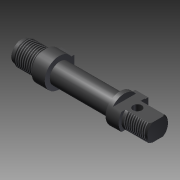
# Autodesk Inventor part: 16N2A12A010-(N0-cilindro)
Saved by Autodesk Inventor 2011 SP1 (Build 150282100, 282)
## iProperties
Created: 2018-01-08
Part Number: 16N2A12A010-(N0-cilindro)
Catalog Web Link: www.cadenas.de
Description: Minicylinders Serie 16 - 24 - 25 Single and double acting  Cetop RP52-P DIN/ISO 6432-Cylinder-
Vendor: CAMOZZI
Document SubType Name: Modeling
Designer: psAdmin
Manufacturer: CAMOZZI
Mass: 14.7107 g
Surface Area: 75.8728 cm^2
Volume: 14.7107 cm^3
Density: 1 g/cm^3
Category: PARTsolutions
Company: CAMOZZI
Title: 16N2A12A010
Author: Cadenas PARTsolutions
PSOL_IDENT_0: {$CADENAS_DATA\23d-libs\camozzi\movimento\cilindri_a_norma_e_cilindri_standard\minicilindri_serie_16
PSOL_IDENT_1: _24_25\minicilindr_serie_16_24_25_cilindro.prj},289 {VTYP=3D},{NB=16N2A12A010-(N0-cilindro)},{LINA=1
PSOL_IDENT_2: 6N2A12A010},{NN=Minicylinders Serie 16 - 24 - 25 Single and double acting  Cetop RP52-P DIN/ISO 6432
PSOL_IDENT_3: -Cylinder},{DATE=27.07.2017 08:45:31},{GEOMDATE=02.04.2015 14:04:54},{VERSION=},{LINEID=40},{LINESUB
PSOL_IDENT_4: ID=-1},{WBVAR=FUNZ,HUBT,HUB,TYP,LSTELO}  {NB=16N2A12A010-(N0-cilindro)},{LINA=16N2A12A010},{KT=DUMMY
PSOL_IDENT_5: },{IDNR=},{SERIE=16},{PHY=12},{EW=12},{KW=8},{BE=M16x1.5},{BENDM=16.000},{BEKDM=14.160},{KK=M6x1},{K
PSOL_IDENT_6: KNDM=6.000},{KKDM=4.773},{CD=6},{VERSION=N = standard},{FUNZ=2},{HUBT=N},{HUB=10},{MAT=A = stelo INO
PSOL_IDENT_7: X rullato - camicia inox},{TYP=A},{V=V = guarnizione stelo viton},{LSTELO=0},{LSTELOX=[0-1000]},{D1=
PSOL_IDENT_8: 14.0},{EE=M5},{EENDM=5.000},{EEKDM=4.019},{D2=6},{L1=105.0},{L11=105.0},{L12=126.0},{L13=0.000},{XC=
PSOL_IDENT_9: 75},{XC1=75},{XC2=0.000},{L2=50.0},{AM=16},{L3=15},{L4=4.5},{L5=17},{L5X1=17},{L5X2=0.000},{L=9},{WF=
PSOL_IDENT_10: 22},{WF1=22},{WF2=0.000},{L6=9},{L7=38},{L7X1=38},{L7X2=0.000},{KV=24},{SW=5},{D=20.5},{D3=20},{HUBA=
PSOL_IDENT_11: -},{FIN=1,'1=semplice effetto',2,'2=doppio effetto',3,'3=doppio effetto stelo passante',7,'7=s.e. st
PSOL_IDENT_12: elo passante'},{HUBIN=10,25,40,50,80,100,125,160,200,250,300},{HUBIN1=10,25,40,50},{HUBIN2=[10:50]},
PSOL_IDENT_13: {HUBIN3=10,25,40,50,80,100,125,160,200,250,300},{HUBIN4=[10:300]},{TYPIN1= 'A', 'A=ghiera V + dado s
PSOL_IDENT_14: telo U'},{TYPIN2= 'A', 'A=ghiera V + dado stelo U'},{TYPIN= 'A', 'A=ghiera V + dado stelo U'},{L51=2
PSOL_IDENT_15: .000},{PRA=1},{HUBX=010},{PHYX=12},{XS=0.000},{YS=0.000},{TB=0.000},{TS=0.000},{DS=0.000}
NN: Minicylinders Serie 16 - 24 - 25 Single and double acting  Cetop RP52-P DIN/ISO 6432-Cylinder
NB: 16N2A12A010-(N0-cilindro)
NBSYN: $SERIE.N$FUNZ.A$PHYX.$TYP.$HUBX.-($HUBT.$LSTELO.-cilindro)
LINA: 16N2A12A010
SERIE: 16
PHY: 12
EW: 12
KW: 8
BE: M16x1.5
KK: M6x1
CD: 6
VERSION: N = standard
FUNZ: 2=doppio effetto
HUBT: standard
HUB: 10
MAT: A = stelo INOX rullato - camicia inox
TYP: A=ghiera V + dado stelo U
V: V = guarnizione stelo viton
LSTELO: 0
D1: 14.0
EE: M5
D2: 6
L1: 105.0
L13: 0.000
XC1: 75
XC2: 0.000
L2: 50.0
AM: 16
L3: 15
L4: 4.5
L5X1: 17
L5X2: 0.000
L: 9
WF1: 22
WF2: 0.000
L6: 9
L7X1: 38
L7X2: 0.000
KV: 24
SW: 5
D: 20.5
D3: 20
HUBA: -
TYPIN1: 'A', 'A=ghiera V + dado stelo U'
TYPIN2: 'A', 'A=ghiera V + dado stelo U'
L51: 2.000
XS: 0.000
YS: 0.000
TB: 0.000
TS: 0.000
DS: 0.000
SUPPLIER: CAMOZZI
ARTICLENO: 16N2A12A010-(N0-cilindro)
BOMINFO: 16N2A12A010
CREATOR: CADENAS GmbH
Autodesk Inventor part; units mm, degrees
sketch "Skizze_1" plane through (0, 0, 0) normal (0, 0, 1) x (1, 0, 0)
  line L0 (77, 0) -> (-17, 0)
  line L1 (-17, 0) -> (-17, 7.08)
  line L2 (-17, 7.08) -> (-15, 7.08)
  line L3 (-15, 7.08) -> (-14.08, 8)
  line L4 (-14.08, 8) -> (0, 8)
  line L5 (0, 8) -> (0, 10)
  line L6 (0, 10) -> (9, 10)
  line L7 (9, 10) -> (9, 6.5)
  line L8 (9, 6.5) -> (9.5, 7)
  line L9 (9.5, 7) -> (50.5, 7)
  line L10 (50.5, 7) -> (51, 6.5)
  line L11 (51, 6.5) -> (51, 10)
  line L12 (51, 10) -> (60, 10)
  line L13 (60, 10) -> (60, 8)
  line L14 (60, 8) -> (76.08, 8)
  line L15 (76.08, 8) -> (77, 7.08)
  line L16 (77, 7.08) -> (77, 0)
  line L17 (77, 0) -> (-17, 0)
  constraints: 36 end point
revolve "Revolution1" add sketch "Skizze_1" angle 360 about axis through (77, 0, 0) along (1, 0, 0)
thread "Thread1" size "M16x1.5" class "6g" standard "ISO Metric profile" length 12.08
thread "Thread2" size "M16x1.5" class "6g" standard "ISO Metric profile" length 14.4865
sketch "Skizze_3" plane through (0, 0, 0) normal (1, 0, 0) x (0, 1, 0)
  line L0 (10.5, 5.5) -> (0, 5.5)
  line L1 (0, 5.5) -> (0, -5.5)
  line L2 (0, -5.5) -> (10.5, -5.5)
  line L3 (10.5, -5.5) -> (10.5, 5.5)
  constraints: 8 end point
extrude "Extrusion1" add sketch "Skizze_3" along normal blind 9
sketch "Skizze_4" plane through (60, 0, 0) normal (1, 0, 0) x (0, 0, -1)
  line L0 (-5.5, 10.5) -> (-5.5, 0)
  line L1 (-5.5, 0) -> (5.5, 0)
  line L2 (5.5, 0) -> (5.5, 10.5)
  line L3 (5.5, 10.5) -> (-5.5, 10.5)
  constraints: 8 end point
extrude "Extrusion2" add sketch "Skizze_4" against normal blind 9
sketch "Skizze_16_ALT_Drilling_1" plane through (0, 0, 0) normal (0, 0, 1) x (1, 0, 0)
  line L0 (51, 0) -> (-17, 0)
  line L1 (-17, 0) -> (-17, 3)
  line L2 (-17, 3) -> (38, 3)
  line L3 (38, 3) -> (38, 5.6)
  line L4 (38, 5.6) -> (51, 5.6)
  line L5 (51, 5.6) -> (51, 0)
  line L6 (51, 0) -> (-17, 0)
  constraints: 14 end point
revolve "Revolution2" cut sketch "Skizze_16_ALT_Drilling_1" angle 360 about axis through (51, 0, 0) along (1, 0, 0)
sketch "Skizze_7" plane through (0, 0, 0) normal (0, 1, 0) x (-1, 0, 0)
  line L0 (-54, -12) -> (-54, -6)
  line L1 (-54, -6) -> (-77, -6)
  line L2 (-77, -6) -> (-77, 6)
  line L3 (-77, 6) -> (-54, 6)
  line L4 (-54, 6) -> (-54, 12)
  line L5 (-54, 12) -> (-86, 12)
  line L6 (-86, 12) -> (-86, -12)
  line L7 (-86, -12) -> (-54, -12)
  constraints: 16 end point
extrude "Extrusion3" cut sketch "Skizze_7" along normal mid plane 24
sketch "Skizze_8" plane through (0, 0, 0) normal (0, 0, 1) x (1, 0, 0)
  circle A0 centre (63, 0) radius 3
  constraints: 1 centre point
extrude "Extrusion4" cut sketch "Skizze_8" along normal mid plane 24
sketch "Skizze_9_ALT_Drilling_2" plane through (0, 0, 0) normal (0, 0, 1) x (1, 0, 0)
  line L0 (4.5, 10.5) -> (4.5, 5.3398)
  line L1 (4.5, 5.3398) -> (2.4905, 6.5)
  line L2 (2.4905, 6.5) -> (2.4905, 10.0095)
  line L3 (2.4905, 10.0095) -> (2, 10.5)
  line L4 (2, 10.5) -> (4.5, 10.5)
  line L5 (4.5, 10.5) -> (4.5, 5.3398)
  constraints: 12 end point
revolve "Revolution3" cut sketch "Skizze_9_ALT_Drilling_2" angle 360 about axis through (4.5, 10.5, 0) along (0, 1, 0)
sketch "Skizze_10_ALT_Drilling_3" plane through (0, 0, 0) normal (0, 0, 1) x (1, 0, 0)
  line L0 (55.5, 10.5) -> (55.5, 5.3398)
  line L1 (55.5, 5.3398) -> (53.4905, 6.5)
  line L2 (53.4905, 6.5) -> (53.4905, 10.0095)
  line L3 (53.4905, 10.0095) -> (53, 10.5)
  line L4 (53, 10.5) -> (55.5, 10.5)
  line L5 (55.5, 10.5) -> (55.5, 5.3398)
  constraints: 12 end point
revolve "Revolution4" cut sketch "Skizze_10_ALT_Drilling_3" angle 360 about axis through (55.5, 10.5, 0) along (0, 1, 0)
ref_plane "C1_XY" through (0, 0, 0) normal (1, 0, 0) x (0, 0, -1)
ref_plane "C1_YZ" through (0, 0, 0) normal (0, 0, -1) x (0, 1, 0)
ref_plane "C1_ZX" through (0, 0, 0) normal (0, 1, 0) x (1, 0, 0)
ref_plane "CD1_XY" through (0, 0, 0) normal (1, 0, 0) x (0, 0, -1)
ref_plane "CD1_YZ" through (0, 0, 0) normal (0, 0, -1) x (0, 1, 0)
ref_plane "CD1_ZX" through (0, 0, 0) normal (0, 1, 0) x (1, 0, 0)
ref_plane "CD2_XY" through (60, 0, 0) normal (1, 0, 0) x (0, 0, -1)
ref_plane "CD2_YZ" through (60, 0, 0) normal (0, 0, -1) x (0, 1, 0)
ref_plane "CD2_ZX" through (60, 0, 0) normal (0, 1, 0) x (1, 0, 0)
ref_plane "RL_XY" through (-17, 0, 0) normal (1, 0, 0) x (0, 0, -1)
ref_plane "RL_YZ" through (-17, 0, 0) normal (0, 0, -1) x (0, 1, 0)
ref_plane "RL_ZX" through (-17, 0, 0) normal (0, 1, 0) x (1, 0, 0)
body "Solid1"
